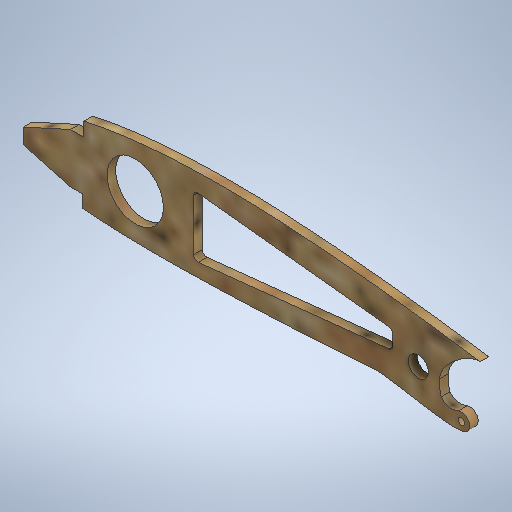
# Autodesk Inventor part: 2414 basic aerofoil
Saved by Autodesk Inventor 2025.1 (Build 291241000, 241)
## iProperties
Created: 2024-11-04
Part Number: 2414 basic aerofoil
Material: Generic
Document SubType Name: Modeling
Designer: johan
Density: 1 g/cm^3
Appearance: Default
Author: johan
Autodesk Inventor part; units mm, degrees
ref_plane "YZ Plane" through (0, 0, 0) normal (1, 0, 0) x (0, 1, 0)
ref_plane "XZ Plane" through (0, 0, 0) normal (0, 1, 0) x (-1, 0, 0)
ref_plane "XY Plane" through (0, 0, 0) normal (0, 0, 1) x (1, 0, 0)
sketch "Sketch3" plane through (0, 0, 0) normal (0, 0, 1) x (1, 0, 0)
  circle A0 centre (229.65, -11.9427) radius 1.5
  spline S0 degree 4 poles (238.1757, 16.0311) (233.8653, 16.6929) (224.6025, 10.7643) (219.5956, 4.5835) (219.6501, -0.0623) knots 0 0 0 0 0 1 1 1 1 1
  line L0 (219.65, 0.0573) -> (219.65, -15.4427) construction
  line L1 (219.65, -15.4427) -> (229.65, -15.4427) construction
  spline S1 degree 2 poles (219.65, 0.0573) (219.65, -15.4427) (229.65, -15.4427) knots 1 1 1 2 2 2
  spline S2 degree 4 poles (229.65, -15.4427) (232.2479, -15.4427) (236.4672, -15.0793) (240.4055, -14.6746) (252.3645, -10.2234) (260.9514, -5.3859) (262.6121, -5.8597) (266.6898, -4.9446) knots 0 0 0 0 0 0.251889 0.432474 0.605523 1 1 1 1 1
  circle A1 centre (229.65, 0.0573) radius 2.5
  line L2 (248.053, 14.4852) -> (228.2984, 17.5771) construction
  arc A2 (246.0728, 14.7656) -> (230.2696, 17.2391) centre (68.4762, -1068.2032) ccw construction
  spline S3 degree 4 poles (266.6898, -4.9446) (271.994, -4.4741) (279.0613, -3.8343) (287.5875, -3.0546) (296.9098, -2.171) (302.7209, -1.6224) (307.605, -1.1306) (311.8361, -0.7493) (314.775, -0.3922) (317.509, -0.2216) (318.5616, 0.026) (320.2917, 0.0146) (318.5753, 0.2326) (317.5642, 0.6172) (314.8742, 1.1425) (312.0031, 1.8752) (307.848, 2.7857) (303.0522, 3.8732) (297.3328, 5.1077) (290.8741, 6.4737) (283.6458, 7.946) (275.7215, 9.5026) (267.1347, 11.1189) (256.7523, 12.9847) (248.2675, 14.4211) (242.0067, 15.4315) (238.1757, 16.0311) knots 0 0 0 0 0 0.127872 0.175449 0.220295 0.262069 0.300363 0.334656 0.364212 0.387684 0.40612 0.423013 0.44145 0.464926 0.494492 0.528803 0.567125 0.608942 0.653849 0.701506 0.751617 0.803914 0.85815 0.914094 1 1 1 1 1
  line L3 (225.208, -15.4427) -> (234.092, -15.4427) construction
  arc A3 (226.1087, -15.2948) -> (233.1912, -15.2948) centre (229.65, 27.0439) ccw construction
  line L4 (238.1757, 16.0311) -> (233.8653, 16.6929) construction
  line L5 (233.8653, 16.6929) -> (224.6025, 10.7643) construction
  line L6 (224.6025, 10.7643) -> (219.5956, 4.5835) construction
  line L7 (219.5956, 4.5835) -> (219.6501, -0.0623) construction
  point P0 (0, 0)
  point P1 (319.65, 0.0573)
  point P2 (319.1928, 0.1662)
  point P3 (317.8239, 0.4911)
  point P4 (315.5508, 1.0254)
  point P5 (312.3867, 1.7598)
  point P6 (308.3496, 2.6802)
  point P7 (303.4629, 3.7707)
  point P8 (297.7548, 5.0118)
  point P9 (291.2586, 6.3828)
  point P10 (284.0121, 7.8612)
  point P11 (276.0585, 9.4236)
  point P12 (267.4446, 11.046)
  point P13 (258.222, 12.7041)
  point P14 (248.4459, 14.3739)
  point P15 (283.4097, -3.4332)
  point P16 (290.7465, -2.7525)
  point P17 (297.3372, -2.1309)
  point P18 (303.1389, -1.575)
  point P19 (308.1141, -1.0914)
  point P20 (312.2304, -0.6861)
  point P21 (315.4602, -0.3648)
  point P22 (317.7828, -0.1314)
  point P23 (319.1823, 0.0099)
  point P24 (220.8549, -8.8358)
  point P25 (235.9469, -15.0689)
  point P26 (241.1681, -14.0895)
  point P27 (249.8679, -10.9203)
  point P28 (258.2267, -7.1402)
  point P29 (262.2449, -5.8127)
  dimension "d24" = 3
  dimension "d25" = 5
  constraints: 4 centre point, 4 end point, 4 midpoint, 2 point on circle, 1 collinear, 1 horizontal, 45 other
  measures "d24" diameter of A0
  measures "d25" diameter of A1
sketch "Sketch2" plane through (0, 0, 0) normal (0, 0, 1) x (1, 0, 0)
  circle A0 centre (79.5236, 4.6493) radius 12.9985
  line L0 (79.5236, 4.6493) -> (79.5236, 24.6629) construction
  circle A1 centre (209.8094, 0) radius 4.6445
  line L1 (79.5236, 4.6493) -> (209.6459, 4.6493) construction
  line L2 (319.8094, 1.4096) -> (219.8094, 1.4096) construction
  line L3 (219.8094, 18.7497) -> (219.8094, -8.9327) construction
  line L4 (106.3751, 16.4243) -> (106.3751, -7.1256)
  line L5 (198.1034, 7.0516) -> (198.1034, 2.247)
  line L6 (196.3158, 0.2584) -> (108.5875, -9.1143)
  line L7 (108.5875, 18.413) -> (196.3158, 9.0403)
  arc A2 (108.5875, 18.413) -> (106.3751, 16.4243) centre (108.3751, 16.4243) ccw
  arc A3 (106.3751, -7.1256) -> (108.5875, -9.1143) centre (108.3751, -7.1256) ccw
  arc A4 (196.3158, 0.2584) -> (198.1034, 2.247) centre (196.1034, 2.247) ccw
  arc A5 (198.1034, 7.0516) -> (196.3158, 9.0403) centre (196.1034, 7.0516) ccw
  spline S0 degree 4 poles (238.1757, 16.0311) (233.8653, 16.6929) (224.6025, 10.7643) (219.5956, 4.5835) (219.6501, -0.0623) knots 0 0 0 0 0 1 1 1 1 1
  arc A6 (230.4778, -15.6002) -> (228.2648, -8.4579) centre (229.65, -11.9427) ccw
  line L8 (230.4778, -15.6002) -> (222.25, -17.4625) construction
  line L9 (222.25, -17.4625) -> (195.7966, -10.4606) construction
  line L10 (195.7966, -10.4606) -> (188.9868, -11.1932) construction
  spline S1 degree 3 poles (230.4778, -15.6002) (222.25, -17.4625) (195.7966, -10.4606) (188.9868, -11.1932) knots 1 1 1 1 2 2 2 2
  circle A7 centre (229.65, -11.9427) radius 1.5
  line L11 (220.3053, -6.8627) -> (223.2264, -10.4606) construction
  line L12 (223.2264, -10.4606) -> (228.2648, -8.4579) construction
  spline S2 degree 2 poles (220.3053, -6.8627) (223.2264, -10.4606) (228.2648, -8.4579) knots 1 1 1 2 2 2
  spline S3 degree 4 poles (238.1745, 16.0313) (235.5132, 16.4439) (231.7878, 17.0257) (226.8733, 17.74) (220.8632, 18.6092) (216.3883, 19.2219) (211.8661, 19.8192) (207.3172, 20.4094) (202.7175, 20.9784) (198.0904, 21.5322) (193.4308, 22.0659) (188.7476, 22.5786) (184.0434, 23.0697) (179.3239, 23.537) (174.5933, 23.9807) (169.8563, 24.3963) (165.1181, 24.7863) (160.3834, 25.1464) (155.6559, 25.4767) (150.9421, 25.7763) (146.2406, 26.0437) (141.5663, 26.2773) (136.8929, 26.4777) (132.2373, 26.6298) (127.6183, 26.7376) (123.0377, 26.7984) (118.5026, 26.8126) (114.0193, 26.7799) (109.5903, 26.6995) (105.2253, 26.5724) (100.9175, 26.3997) (96.6993, 26.1753) (92.5176, 25.9171) (88.5501, 25.5865) (84.3125, 25.2786) (81.0633, 24.7646) (76.6043, 24.424) (73.0877, 23.9033) (69.3817, 23.3842) (65.8759, 22.8129) (62.4567, 22.2097) (59.1589, 21.5685) (55.9715, 20.8934) (52.9021, 20.1858) (49.9535, 19.4467) (47.1274, 18.6788) (44.4279, 17.8843) (41.8573, 17.0635) (39.4171, 16.2211) (37.1113, 15.3565) (34.9402, 14.4741) (32.9073, 13.5735) (31.0136, 12.6584) (29.2606, 11.7303) (27.6501, 10.79) (26.1834, 9.8406) (24.8609, 8.8829) (23.6848, 7.9176) (22.654, 6.9484) (21.7717, 5.9692) (21.0345, 4.9988) (20.4521, 3.9916) (19.9895, 3.0305) (19.7297, 1.8193) (19.5077, 1.2694) (19.9773, -1.5998) (20.0391, -1.5907) (20.6304, -2.8993) (21.2091, -3.6295) (21.976, -4.5261) (22.8733, -5.32) (23.921, -6.1177) (25.1038, -6.8705) (26.4262, -7.5981) (27.8839, -8.2925) (29.4774, -8.9572) (31.2033, -9.5906) (33.0618, -10.1918) (35.0491, -10.7623) (37.1643, -11.3005) (39.4051, -11.8066) (41.7689, -12.2803) (44.2534, -12.722) (46.8564, -13.1312) (49.5754, -13.507) (52.4069, -13.8511) (55.3492, -14.1625) (58.3987, -14.4423) (61.5532, -14.6896) (64.8087, -14.906) (68.1633, -15.0908) (71.6131, -15.2459) (75.155, -15.3704) (78.7859, -15.4669) (82.5025, -15.5344) (86.3016, -15.575) (90.1791, -15.589) (94.132, -15.5779) (98.1568, -15.5431) (102.2497, -15.4847) (106.4069, -15.4055) (110.6252, -15.3059) (114.8998, -15.1867) (119.2282, -15.0511) (123.6052, -14.8989) (128.0281, -14.7321) (132.495, -14.5521) (136.999, -14.3599) (141.5497, -14.1602) (146.1548, -13.9405) (150.7789, -13.7048) (155.427, -13.4523) (160.0929, -13.1848) (164.7606, -12.9057) (169.4585, -12.6088) (174.1166, -12.316) (179.6377, -11.9145) (183.4005, -11.7398) (187.2013, -11.3114) (188.9868, -11.1932) knots 0 0 0 0 0 0.024474 0.034359 0.044305 0.054303 0.064353 0.074444 0.08457 0.094728 0.104914 0.115121 0.125345 0.135581 0.145823 0.156067 0.166308 0.17654 0.186758 0.196958 0.207141 0.217307 0.227451 0.237569 0.247647 0.257677 0.267653 0.27757 0.287423 0.297207 0.306917 0.316547 0.326093 0.335424 0.344778 0.354034 0.363182 0.372345 0.381273 0.390078 0.398756 0.407301 0.415708 0.423971 0.432085 0.440043 0.44784 0.45547 0.462928 0.470207 0.477303 0.484208 0.490919 0.497431 0.503739 0.50984 0.515732 0.521417 0.526898 0.532184 0.537287 0.542231 0.547048 0.552443 0.557443 0.562445 0.56749 0.571956 0.576896 0.581992 0.587264 0.592728 0.59839 0.604255 0.610321 0.616588 0.623052 0.629708 0.636553 0.643581 0.650786 0.658162 0.665705 0.673407 0.681264 0.689271 0.69742 0.705708 0.714128 0.722676 0.731346 0.740132 0.74903 0.758035 0.767142 0.776346 0.785641 0.795024 0.804488 0.81403 0.823645 0.833327 0.843073 0.852877 0.862734 0.872641 0.882596 0.892602 0.902655 0.912749 0.922875 0.93302 0.94318 0.95335 0.963525 0.973699 0.98409 1 1 1 1 1
  line L13 (28.0161, 4.4987) -> (28.0161, -2.5013)
  line L14 (19.6371, 1.026) -> (319.5749, 0.0498) construction
  line L15 (28.0161, -2.5013) -> (49.7201, -8.4902)
  line L16 (28.0161, 4.4987) -> (49.7201, 14.4201)
  line L17 (55.296, -14.1484) -> (55.296, -8.4902)
  line L18 (55.296, -8.4902) -> (49.7201, -8.4902)
  line L19 (55.9195, 20.8697) -> (55.9195, 14.4201)
  line L20 (55.9195, 14.4201) -> (49.7201, 14.4201)
  line L21 (238.1745, 16.0313) -> (235.5132, 16.4439) construction
  line L22 (235.5132, 16.4439) -> (231.7878, 17.0257) construction
  line L23 (231.7878, 17.0257) -> (226.8733, 17.74) construction
  line L24 (226.8733, 17.74) -> (220.8632, 18.6092) construction
  line L25 (220.8632, 18.6092) -> (216.3883, 19.2219) construction
  line L26 (216.3883, 19.2219) -> (211.8661, 19.8192) construction
  line L27 (211.8661, 19.8192) -> (207.3172, 20.4094) construction
  line L28 (207.3172, 20.4094) -> (202.7175, 20.9784) construction
  line L29 (202.7175, 20.9784) -> (198.0904, 21.5322) construction
  line L30 (198.0904, 21.5322) -> (193.4308, 22.0659) construction
  line L31 (193.4308, 22.0659) -> (188.7476, 22.5786) construction
  line L32 (188.7476, 22.5786) -> (184.0434, 23.0697) construction
  line L33 (184.0434, 23.0697) -> (179.3239, 23.537) construction
  line L34 (179.3239, 23.537) -> (174.5933, 23.9807) construction
  line L35 (174.5933, 23.9807) -> (169.8563, 24.3963) construction
  line L36 (169.8563, 24.3963) -> (165.1181, 24.7863) construction
  line L37 (165.1181, 24.7863) -> (160.3834, 25.1464) construction
  line L38 (160.3834, 25.1464) -> (155.6559, 25.4767) construction
  line L39 (155.6559, 25.4767) -> (150.9421, 25.7763) construction
  line L40 (150.9421, 25.7763) -> (146.2406, 26.0437) construction
  line L41 (146.2406, 26.0437) -> (141.5663, 26.2773) construction
  line L42 (141.5663, 26.2773) -> (136.8929, 26.4777) construction
  line L43 (136.8929, 26.4777) -> (132.2373, 26.6298) construction
  line L44 (132.2373, 26.6298) -> (127.6183, 26.7376) construction
  line L45 (127.6183, 26.7376) -> (123.0377, 26.7984) construction
  line L46 (123.0377, 26.7984) -> (118.5026, 26.8126) construction
  line L47 (118.5026, 26.8126) -> (114.0193, 26.7799) construction
  line L48 (114.0193, 26.7799) -> (109.5903, 26.6995) construction
  line L49 (109.5903, 26.6995) -> (105.2253, 26.5724) construction
  line L50 (105.2253, 26.5724) -> (100.9175, 26.3997) construction
  line L51 (100.9175, 26.3997) -> (96.6993, 26.1753) construction
  line L52 (96.6993, 26.1753) -> (92.5176, 25.9171) construction
  line L53 (92.5176, 25.9171) -> (88.5501, 25.5865) construction
  line L54 (88.5501, 25.5865) -> (84.3125, 25.2786) construction
  line L55 (84.3125, 25.2786) -> (81.0633, 24.7646) construction
  line L56 (81.0633, 24.7646) -> (76.6043, 24.424) construction
  line L57 (76.6043, 24.424) -> (73.0877, 23.9033) construction
  line L58 (73.0877, 23.9033) -> (69.3817, 23.3842) construction
  line L59 (69.3817, 23.3842) -> (65.8759, 22.8129) construction
  line L60 (65.8759, 22.8129) -> (62.4567, 22.2097) construction
  line L61 (62.4567, 22.2097) -> (59.1589, 21.5685) construction
  line L62 (59.1589, 21.5685) -> (55.9715, 20.8934) construction
  line L63 (55.9715, 20.8934) -> (52.9021, 20.1858) construction
  line L64 (52.9021, 20.1858) -> (49.9535, 19.4467) construction
  line L65 (49.9535, 19.4467) -> (47.1274, 18.6788) construction
  line L66 (47.1274, 18.6788) -> (44.4279, 17.8843) construction
  line L67 (44.4279, 17.8843) -> (41.8573, 17.0635) construction
  line L68 (41.8573, 17.0635) -> (39.4171, 16.2211) construction
  line L69 (39.4171, 16.2211) -> (37.1113, 15.3565) construction
  line L70 (37.1113, 15.3565) -> (34.9402, 14.4741) construction
  line L71 (34.9402, 14.4741) -> (32.9073, 13.5735) construction
  line L72 (32.9073, 13.5735) -> (31.0136, 12.6584) construction
  line L73 (31.0136, 12.6584) -> (29.2606, 11.7303) construction
  line L74 (29.2606, 11.7303) -> (27.6501, 10.79) construction
  line L75 (27.6501, 10.79) -> (26.1834, 9.8406) construction
  line L76 (26.1834, 9.8406) -> (24.8609, 8.8829) construction
  line L77 (24.8609, 8.8829) -> (23.6848, 7.9176) construction
  line L78 (23.6848, 7.9176) -> (22.654, 6.9484) construction
  line L79 (22.654, 6.9484) -> (21.7717, 5.9692) construction
  line L80 (21.7717, 5.9692) -> (21.0345, 4.9988) construction
  line L81 (21.0345, 4.9988) -> (20.4521, 3.9916) construction
  line L82 (20.4521, 3.9916) -> (19.9895, 3.0305) construction
  line L83 (19.9895, 3.0305) -> (19.7297, 1.8193) construction
  line L84 (19.7297, 1.8193) -> (19.5077, 1.2694) construction
  line L85 (19.5077, 1.2694) -> (19.9773, -1.5998) construction
  line L86 (19.9773, -1.5998) -> (20.0391, -1.5907) construction
  line L87 (20.0391, -1.5907) -> (20.6304, -2.8993) construction
  line L88 (20.6304, -2.8993) -> (21.2091, -3.6295) construction
  line L89 (21.2091, -3.6295) -> (21.976, -4.5261) construction
  line L90 (21.976, -4.5261) -> (22.8733, -5.32) construction
  line L91 (22.8733, -5.32) -> (23.921, -6.1177) construction
  line L92 (23.921, -6.1177) -> (25.1038, -6.8705) construction
  line L93 (25.1038, -6.8705) -> (26.4262, -7.5981) construction
  line L94 (26.4262, -7.5981) -> (27.8839, -8.2925) construction
  line L95 (27.8839, -8.2925) -> (29.4774, -8.9572) construction
  line L96 (29.4774, -8.9572) -> (31.2033, -9.5906) construction
  line L97 (31.2033, -9.5906) -> (33.0618, -10.1918) construction
  line L98 (33.0618, -10.1918) -> (35.0491, -10.7623) construction
  line L99 (35.0491, -10.7623) -> (37.1643, -11.3005) construction
  line L100 (37.1643, -11.3005) -> (39.4051, -11.8066) construction
  line L101 (39.4051, -11.8066) -> (41.7689, -12.2803) construction
  line L102 (41.7689, -12.2803) -> (44.2534, -12.722) construction
  line L103 (44.2534, -12.722) -> (46.8564, -13.1312) construction
  line L104 (46.8564, -13.1312) -> (49.5754, -13.507) construction
  line L105 (49.5754, -13.507) -> (52.4069, -13.8511) construction
  line L106 (52.4069, -13.8511) -> (55.3492, -14.1625) construction
  line L107 (55.3492, -14.1625) -> (58.3987, -14.4423) construction
  line L108 (58.3987, -14.4423) -> (61.5532, -14.6896) construction
  line L109 (61.5532, -14.6896) -> (64.8087, -14.906) construction
  line L110 (64.8087, -14.906) -> (68.1633, -15.0908) construction
  line L111 (68.1633, -15.0908) -> (71.6131, -15.2459) construction
  line L112 (71.6131, -15.2459) -> (75.155, -15.3704) construction
  line L113 (75.155, -15.3704) -> (78.7859, -15.4669) construction
  line L114 (78.7859, -15.4669) -> (82.5025, -15.5344) construction
  line L115 (82.5025, -15.5344) -> (86.3016, -15.575) construction
  line L116 (86.3016, -15.575) -> (90.1791, -15.589) construction
  line L117 (90.1791, -15.589) -> (94.132, -15.5779) construction
  line L118 (94.132, -15.5779) -> (98.1568, -15.5431) construction
  line L119 (98.1568, -15.5431) -> (102.2497, -15.4847) construction
  line L120 (102.2497, -15.4847) -> (106.4069, -15.4055) construction
  line L121 (106.4069, -15.4055) -> (110.6252, -15.3059) construction
  line L122 (110.6252, -15.3059) -> (114.8998, -15.1867) construction
  line L123 (114.8998, -15.1867) -> (119.2282, -15.0511) construction
  line L124 (119.2282, -15.0511) -> (123.6052, -14.8989) construction
  line L125 (123.6052, -14.8989) -> (128.0281, -14.7321) construction
  line L126 (128.0281, -14.7321) -> (132.495, -14.5521) construction
  line L127 (132.495, -14.5521) -> (136.999, -14.3599) construction
  line L128 (136.999, -14.3599) -> (141.5497, -14.1602) construction
  line L129 (141.5497, -14.1602) -> (146.1548, -13.9405) construction
  line L130 (146.1548, -13.9405) -> (150.7789, -13.7048) construction
  line L131 (150.7789, -13.7048) -> (155.427, -13.4523) construction
  line L132 (155.427, -13.4523) -> (160.0929, -13.1848) construction
  line L133 (160.0929, -13.1848) -> (164.7606, -12.9057) construction
  line L134 (164.7606, -12.9057) -> (169.4585, -12.6088) construction
  line L135 (169.4585, -12.6088) -> (174.1166, -12.316) construction
  line L136 (174.1166, -12.316) -> (179.6377, -11.9145) construction
  line L137 (179.6377, -11.9145) -> (183.4005, -11.7398) construction
  line L138 (183.4005, -11.7398) -> (187.2013, -11.3114) construction
  line L139 (187.2013, -11.3114) -> (188.9868, -11.1932) construction
  arc A8 (219.65, 0.0573) -> (220.3053, -6.8627) centre (237.2502, -1.767) ccw
  line L140 (19.6371, 1.026) -> (319.6371, 0.9101)
  line L141 (319.6371, 0.9101) -> (19.6372, 1.026)
  point P0 (0, 0)
  point P1 (319.5767, 0.0747)
  point P2 (319.3571, 0.1272)
  point P3 (318.9917, 0.2142)
  point P4 (318.4802, 0.3354)
  point P5 (317.8238, 0.4911)
  point P6 (317.0222, 0.6801)
  point P7 (316.0769, 0.9024)
  point P8 (314.9885, 1.1568)
  point P9 (313.7582, 1.443)
  point P10 (312.3866, 1.7598)
  point P11 (310.8752, 2.1063)
  point P12 (309.2258, 2.4819)
  point P13 (307.4393, 2.8854)
  point P14 (305.5178, 3.3153)
  point P15 (303.4628, 3.7707)
  point P16 (301.2764, 4.2501)
  point P17 (298.9607, 4.7526)
  point P18 (296.5175, 5.2764)
  point P19 (293.9492, 5.8203)
  point P20 (291.2585, 6.3828)
  point P21 (288.4478, 6.9627)
  point P22 (285.5195, 7.5582)
  point P23 (282.4766, 8.1678)
  point P24 (279.3218, 8.79)
  point P25 (276.0584, 9.4236)
  point P26 (272.6891, 10.0668)
  point P27 (269.2175, 10.7178)
  point P28 (265.6469, 11.3757)
  point P29 (261.9803, 12.0381)
  point P30 (258.2219, 12.7041)
  point P31 (254.3747, 13.3722)
  point P32 (250.4426, 14.0403)
  point P33 (246.4295, 14.7072)
  point P34 (242.339, 15.3714)
  point P35 (238.1756, 16.0311)
  point P36 (233.9424, 16.6853)
  point P37 (229.6464, 17.3319)
  point P38 (225.2829, 17.9694)
  point P39 (220.8866, 18.5989)
  point P40 (216.4137, 19.214)
  point P41 (211.8876, 19.8141)
  point P42 (207.3328, 20.4017)
  point P43 (202.7344, 20.9724)
  point P44 (198.1034, 21.5257)
  point P45 (193.4422, 22.0597)
  point P46 (188.7563, 22.5727)
  point P47 (184.0498, 23.0638)
  point P48 (179.3278, 23.5315)
  point P49 (174.5948, 23.9746)
  point P50 (169.8554, 24.391)
  point P51 (165.1148, 24.7804)
  point P52 (160.3775, 25.1407)
  point P53 (155.648, 25.471)
  point P54 (150.9317, 25.7704)
  point P55 (146.2331, 26.0374)
  point P56 (141.557, 26.2708)
  point P57 (136.8821, 26.4682)
  point P58 (132.221, 26.6212)
  point P59 (127.5965, 26.7283)
  point P60 (123.0134, 26.7889)
  point P61 (118.4762, 26.8027)
  point P62 (113.9903, 26.7694)
  point P63 (109.5602, 26.6887)
  point P64 (105.191, 26.5612)
  point P65 (100.8866, 26.3867)
  point P66 (96.6525, 26.1649)
  point P67 (92.4923, 25.8974)
  point P68 (88.4126, 25.5836)
  point P69 (84.4117, 25.2266)
  point P70 (80.9176, 24.8094)
  point P71 (76.6884, 24.3764)
  point P72 (72.962, 23.8901)
  point P73 (69.3404, 23.3611)
  point P74 (65.8205, 22.7937)
  point P75 (62.4085, 22.1882)
  point P76 (59.1069, 21.5462)
  point P77 (52.8493, 20.1605)
  point P78 (49.9, 19.4201)
  point P79 (47.0736, 18.6505)
  point P80 (44.3739, 17.854)
  point P81 (41.8032, 17.032)
  point P82 (39.3636, 16.1872)
  point P83 (37.0581, 15.321)
  point P84 (34.8882, 14.436)
  point P85 (32.8566, 13.5336)
  point P86 (30.9649, 12.6161)
  point P87 (29.2144, 11.6854)
  point P88 (27.607, 10.7431)
  point P89 (26.1443, 9.7914)
  point P90 (24.827, 8.8316)
  point P91 (23.6569, 7.8655)
  point P92 (22.634, 6.8943)
  point P93 (21.7597, 5.9198)
  point P94 (21.0343, 4.943)
  point P95 (20.4583, 3.965)
  point P96 (20.0324, 2.9865)
  point P97 (19.7558, 2.0093)
  point P98 (19.9715, -1.3762)
  point P99 (20.1382, -1.8327)
  point P100 (20.6016, -2.739)
  point P101 (21.209, -3.6146)
  point P102 (21.9605, -4.4616)
  point P103 (22.8548, -5.2795)
  point P104 (23.8911, -6.068)
  point P105 (25.0682, -6.8268)
  point P106 (26.3845, -7.5553)
  point P107 (27.8382, -8.2533)
  point P108 (29.4282, -8.9205)
  point P109 (31.152, -9.5566)
  point P110 (33.0084, -10.1609)
  point P111 (34.9947, -10.7336)
  point P112 (37.1091, -11.2743)
  point P113 (39.3495, -11.7825)
  point P114 (41.7132, -12.2583)
  point P115 (44.1978, -12.7018)
  point P116 (46.8012, -13.1125)
  point P117 (49.5207, -13.4902)
  point P118 (52.353, -13.8355)
  point P119 (58.3467, -14.4293)
  point P120 (61.5021, -14.678)
  point P121 (64.7589, -14.8952)
  point P122 (68.1148, -15.0812)
  point P123 (71.566, -15.2369)
  point P124 (75.1093, -15.3626)
  point P125 (78.7417, -15.4595)
  point P126 (82.4599, -15.5279)
  point P127 (86.2606, -15.569)
  point P128 (90.1399, -15.5837)
  point P129 (94.0945, -15.5732)
  point P130 (98.1211, -15.5387)
  point P131 (102.2158, -15.4811)
  point P132 (106.375, -15.4022)
  point P133 (110.5951, -15.3029)
  point P134 (114.8719, -15.1844)
  point P135 (119.2021, -15.0488)
  point P136 (123.5812, -14.897)
  point P137 (128.0059, -14.7305)
  point P138 (132.4717, -14.5508)
  point P139 (136.9747, -14.3598)
  point P140 (141.5284, -14.1575)
  point P141 (146.1364, -13.9382)
  point P142 (150.7678, -13.7021)
  point P143 (155.419, -13.4498)
  point P144 (160.0852, -13.1828)
  point P145 (164.7616, -12.9023)
  point P146 (169.4443, -12.6098)
  point P147 (174.1283, -12.3059)
  point P148 (178.8092, -11.9924)
  point P149 (183.4817, -11.6699)
  point P150 (192.7877, -11.0037)
  point P151 (202.0079, -10.3149)
  point P152 (206.5748, -9.9645)
  point P153 (211.1069, -9.6117)
  point P154 (215.6, -9.2568)
  point P155 (220.049, -8.9007)
  point P156 (224.4503, -8.5446)
  point P157 (228.7988, -8.1885)
  point P158 (233.0906, -7.8339)
  point P159 (237.3215, -7.4808)
  point P160 (241.4867, -7.1298)
  point P161 (245.5829, -6.7821)
  point P162 (249.6053, -6.4377)
  point P163 (253.5503, -6.0972)
  point P164 (257.4137, -5.7612)
  point P165 (261.1916, -5.4303)
  point P166 (264.8801, -5.1051)
  point P167 (268.4759, -4.7856)
  point P168 (271.9748, -4.4724)
  point P169 (275.3735, -4.1661)
  point P170 (278.6687, -3.867)
  point P171 (281.8565, -3.5757)
  point P172 (284.9345, -3.2925)
  point P173 (287.8985, -3.018)
  point P174 (290.7464, -2.7525)
  point P175 (293.4746, -2.4963)
  point P176 (296.0807, -2.2503)
  point P177 (298.5617, -2.0142)
  point P178 (300.9152, -1.7892)
  point P179 (303.1388, -1.575)
  point P180 (305.2301, -1.3728)
  point P181 (307.1867, -1.1823)
  point P182 (309.0071, -1.0041)
  point P183 (310.6886, -0.8385)
  point P184 (312.2303, -0.6861)
  point P185 (313.6298, -0.5472)
  point P186 (314.8862, -0.4221)
  point P187 (315.9977, -0.3108)
  point P188 (316.9637, -0.2139)
  point P189 (317.7827, -0.1314)
  point P190 (318.4538, -0.0636)
  point P191 (318.9767, -0.0108)
  point P192 (319.3505, 0.027)
  point P193 (28.0161, 0.9987)
  dimension "d9" = 25.997
  dimension "d18" = 9.289
  dimension "d19" = 110
  dimension "d22" = 100
  dimension "d23" = 2
  dimension "d26" = 7.5
  dimension "d38" = 4.6493
  dimension "d42" = 7
  dimension "d43" = 3.5
  dimension "d44" = 30.083
  dimension "d45" = 8.379
  dimension "d50" = 59.8865
  dimension "d52" = 300
  constraints: 36 end point, 12 point on circle, 9 tangent, 8 centre point, 7 vertical, 3 equal radius, 2 coincident, 2 horizontal, 2 perpendicular, 2 point on line, 1 midpoint, 130 other
  measures "d9" diameter of A0
  measures "d18" diameter of A1
  measures "d19" horizontal distance of L2.start A1.centre
  measures "d22" distance of L2.start L2.end
  measures "d23" radius of A2
  measures "d26" diameter of A6
  measures "d38" vertical distance of A1.centre L0.start
  measures "d42" distance of L13.start L13.end
  measures "d43" distance from line of L14 L13.start
  measures "d44" horizontal distance of L15.end L14.start
  measures "d45" horizontal distance of point (28.016, 0.999) L14.start
  measures "d50" horizontal distance of L14.start L0.start
  measures "d52" distance of L14.start L140.end
extrude "Extrusion4" add sketch "Sketch2" along normal blind 4 contours A0 L140 L13 L16 L20 L19 S3 S0 A1 A4 L5 A5 L7 A2 L4 | A0 L140 L4 A3 L6 A4 A1 S0 A8 S2 A6 S1 S3 L17 L18 L15 L13
body "Solid4"
